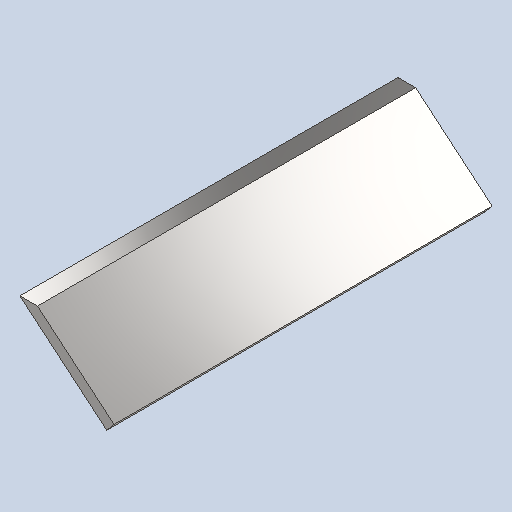
# Autodesk Inventor part: strug
Saved by Autodesk Inventor 2022 (Build 260153000, 153)
## iProperties
Created: 2022-12-26
Part Number: strug
Material: Steel, Alloy
Document SubType Name: Modeling
Designer: Kamil
Density: 7.73 g/cm^3
Appearance: Semi-Polished
Author: Kamil
Autodesk Inventor part; units mm, degrees
ref_plane "YZ Plane" through (0, 0, 0) normal (1, 0, 0) x (0, 1, 0)
ref_plane "XZ Plane" through (0, 0, 0) normal (0, 1, 0) x (-1, 0, 0)
ref_plane "XY Plane" through (0, 0, 0) normal (0, 0, 1) x (1, 0, 0)
sketch "Sketch1" plane through (0, 0, 0) normal (0, 0, 1) x (1, 0, 0)
  line L0 (10.7451, 5.5) -> (50.1922, -27.6) projected
  line L1 (50.1922, -27.6) -> (100, -27.6) projected
  line L2 (100, -27.6) -> (100, -23.6) projected
  line L3 (100, -23.6) -> (83.9, -23.6) projected
  arc A0 (65.8, -5.5) -> (83.9, -23.6) centre (83.9, -5.5) ccw projected
  line L4 (65.8, -5.5) -> (65.8, 5.5) projected
  line L5 (65.8, 5.5) -> (10.7451, 5.5) projected
  line L6 (7.1699, 8.5) -> (10.7451, 5.5) projected
  line L7 (65.8, 5.5) -> (10.7451, 5.5) projected
  line L8 (65.8, 5.5) -> (65.8, 8.5) projected
  line L9 (65.8, 8.5) -> (7.1699, 8.5) projected
  circle A1 centre (83.9, -5.5) radius 16.1 projected
  line L10 (83.9, 10.6) -> (-17.1951, 10.6)
  line L11 (100, -5.5) -> (0, -5.5)
  line L12 (0, -5.5) -> (0, 10.6)
  line L13 (7.1699, 8.5) -> (4.6672, 10.6)
  line L14 (7.1699, 8.5) -> (5.2415, 6.2019)
  line L15 (5.2415, 6.2019) -> (0, 10.6)
  line L16 (0, 10.6) -> (22.9813, -8.6836)
  line L17 (22.9813, -8.6836) -> (24.9097, -6.3855)
  point P0 (0, 0)
  dimension "d0" = 100
  dimension "d1" = 3
  dimension "d2" = 30
  constraints: 16 end point, 4 point on line, 3 perpendicular, 2 horizontal, 2 point on circle, 1 collinear
  measures "d0" distance of L11.start L11.end
  measures "d1" distance of L6.start L14.end
  measures "d2" distance of L12.end L16.end
extrude "Extrusion1" add sketch "Sketch1" against normal blind 100 contours L17 L16 L11 L0 | L11 L16 L14 L6 L0 | L14 L15 L10 L13
body "Solid1"
